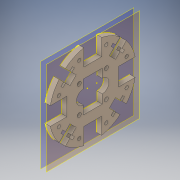
# Autodesk Inventor part: deska
Saved by Autodesk Inventor 2018 (Build 220112000, 112)
## iProperties
Created: 2018-03-10
Part Number: deska
Material: Všeobecné
Document SubType Name: Modeling
Designer: Kuba
Density: 1 g/cm^3
Appearance: Výchozí
Author: Kuba
Autodesk Inventor part; units mm, degrees
ref_plane "YZ Plane" through (0, 0, 0) normal (1, 0, 0) x (0, 1, 0)
ref_plane "XZ Plane" through (0, 0, 0) normal (0, 1, 0) x (-1, 0, 0)
ref_plane "XY Plane" through (0, 0, 0) normal (0, 0, 1) x (1, 0, 0)
sketch "Náčrt1" plane through (0, 0, 0) normal (1, 0, 0) x (0, 1, 0)
  line L0 (19, 6.6) -> (31.312, 6.6)
  line L1 (31.312, -6.6) -> (19, -6.6)
  line L2 (19, -6.6) -> (19, 6.6)
  line L3 (24.8085, 20.2123) -> (16.7938, 12.1976)
  line L4 (16.7938, 12.1976) -> (12.1976, 16.7938)
  line L5 (12.1976, 16.7938) -> (20.2123, 24.8085)
  line L6 (0, 0) -> (14.4957, 14.4957)
  line L7 (6.6, 19) -> (-6.6, 19)
  line L8 (6.6, 31.312) -> (6.6, 19)
  line L9 (-6.6, 19) -> (-6.6, 31.312)
  line L10 (-20.2123, 24.8085) -> (-12.1976, 16.7938)
  line L11 (-12.1976, 16.7938) -> (-16.7938, 12.1976)
  line L12 (-16.7938, 12.1976) -> (-24.8085, 20.2123)
  line L13 (-19, 6.6) -> (-19, -6.6)
  line L14 (-31.312, 6.6) -> (-19, 6.6)
  line L15 (-19, -6.6) -> (-31.312, -6.6)
  line L16 (-24.8085, -20.2123) -> (-16.7938, -12.1976)
  line L17 (-16.7938, -12.1976) -> (-12.1976, -16.7938)
  line L18 (-12.1976, -16.7938) -> (-20.2123, -24.8085)
  line L19 (-6.6, -19) -> (6.6, -19)
  line L20 (-6.6, -31.312) -> (-6.6, -19)
  line L21 (6.6, -19) -> (6.6, -31.312)
  line L22 (20.2123, -24.8085) -> (12.1976, -16.7938)
  line L23 (12.1976, -16.7938) -> (16.7938, -12.1976)
  line L24 (16.7938, -12.1976) -> (24.8085, -20.2123)
  arc A0 (24.8085, -20.2123) -> (31.312, -6.6) centre (0, 0) ccw
  arc A1 (6.6, -31.312) -> (20.2123, -24.8085) centre (0, 0) ccw
  arc A2 (-20.2123, -24.8085) -> (-6.6, -31.312) centre (0, 0) ccw
  arc A3 (-31.312, -6.6) -> (-24.8085, -20.2123) centre (0, 0) ccw
  arc A4 (-24.8085, 20.2123) -> (-31.312, 6.6) centre (0, 0) ccw
  arc A5 (-6.6, 31.312) -> (-20.2123, 24.8085) centre (0, 0) ccw
  arc A6 (31.312, 6.6) -> (24.8085, 20.2123) centre (0, 0) ccw
  arc A7 (20.2123, 24.8085) -> (6.6, 31.312) centre (0, 0) ccw
  line L25 (16.205, 20.8011) -> (20.8011, 16.205)
  line L26 (14.9675, 23.4528) -> (13.5533, 22.0386)
  line L27 (13.5533, 22.0386) -> (22.0386, 13.5533)
  line L28 (22.0386, 13.5533) -> (23.4528, 14.9675)
  line L29 (23.4528, 14.9675) -> (14.9675, 23.4528)
  line L30 (-13.5533, 22.0386) -> (-14.9675, 23.4528)
  line L31 (-22.0386, 13.5533) -> (-13.5533, 22.0386)
  line L32 (-14.9675, 23.4528) -> (-23.4528, 14.9675)
  line L33 (-23.4528, 14.9675) -> (-22.0386, 13.5533)
  line L34 (-22.0386, -13.5533) -> (-23.4528, -14.9675)
  line L35 (-13.5533, -22.0386) -> (-22.0386, -13.5533)
  line L36 (-23.4528, -14.9675) -> (-14.9675, -23.4528)
  line L37 (-14.9675, -23.4528) -> (-13.5533, -22.0386)
  line L38 (13.5533, -22.0386) -> (14.9675, -23.4528)
  line L39 (22.0386, -13.5533) -> (13.5533, -22.0386)
  line L40 (14.9675, -23.4528) -> (23.4528, -14.9675)
  line L41 (23.4528, -14.9675) -> (22.0386, -13.5533)
  point P0 (-14.4957, 14.4957)
  point P1 (-14.4957, -14.4957)
  point P2 (14.4957, -14.4957)
  dimension "d1" = 6.6
  dimension "d2" = 6.6
  dimension "d4" = 6.5
  dimension "d5" = 3.25
  dimension "d6" = 20.5
  dimension "d7" = 45
  dimension "d10" = 360
  dimension "d12" = 2
  dimension "d13" = 12
  dimension "d14" = 1
  dimension "d15" = 2.75
  dimension "d18" = 360
  constraints: 84 end point, 16 point on circle, 8 centre point, 6 midpoint, 4 parallel, 3 perpendicular, 1 coincident, 1 horizontal, 94 other
  measures "d1" vertical distance of point (0, 0) L0.start
  measures "d2" distance from line of point (0, 0) L1
  measures "d4" distance between parallel lines of L3 L5
  measures "d5" distance between parallel lines of L6 L5
  measures "d6" distance from line of point (0, 0) L4
  measures "d7" angle of L2 L6
  measures "d12" distance of L26.start L26.end
  measures "d13" distance of L28.end L26.start
  measures "d14" distance between parallel lines of L25 L29
  measures "d15" distance between parallel lines of L5 L26
extrude "Vysunutí1" add sketch "Náčrt1" along normal mid plane 4 contours L2 L1 A0 L24 L40 L41 L39 L23 L22 L38 A1 L21 L19 L20 A2 L18 L36 L37 L35 L17 L16 L34 A3 L15 L13 L14 A4 L12 L32 L33 L31 L11 L10 L30 A5 L9 L7 L8 A7 L5 L29 L26 L27 L4 L3 L28 A6 L0 | L29 L28 L27 L3 | L5 L27 L26 L29 | L24 L39 L41 L40 | L40 L38 L39 L22 | L32 L30 L31 L10 | L12 L31 L33 L32 | L18 L35 L37 L36 | L36 L34 L35 L16
ref_plane "Pracovní rovina1" through (2, 0, 0) normal (1, 0, 0) x (0, 0, -1)
sketch "Náčrt2" plane through (2, 0, 0) normal (1, 0, 0) x (0, 0, -1)
  line L0 (-6.6, 19) -> (-6.6, 31.312) projected
  arc A0 (-6.6, 31.312) -> (-20.2123, 24.8085) centre (0, 0) ccw projected
  line L1 (-20.2123, 24.8085) -> (-12.1976, 16.7938) projected
  line L2 (-12.1976, 16.7938) -> (-16.7938, 12.1976) projected
  line L3 (-16.7938, 12.1976) -> (-24.8085, 20.2123) projected
  arc A1 (-24.8085, 20.2123) -> (-31.312, 6.6) centre (0, 0) ccw projected
  line L4 (-31.312, 6.6) -> (-19, 6.6) projected
  line L5 (-19, 6.6) -> (-19, -6.6) projected
  line L6 (-19, -6.6) -> (-31.312, -6.6) projected
  arc A2 (-31.312, -6.6) -> (-24.8085, -20.2123) centre (0, 0) ccw projected
  line L7 (-24.8085, -20.2123) -> (-16.7938, -12.1976) projected
  line L8 (-16.7938, -12.1976) -> (-12.1976, -16.7938) projected
  line L9 (-12.1976, -16.7938) -> (-20.2123, -24.8085) projected
  arc A3 (-20.2123, -24.8085) -> (-6.6, -31.312) centre (0, 0) ccw projected
  line L10 (-6.6, -31.312) -> (-6.6, -19) projected
  line L11 (-6.6, -19) -> (6.6, -19) projected
  line L12 (6.6, -19) -> (6.6, -31.312) projected
  arc A4 (6.6, -31.312) -> (20.2123, -24.8085) centre (0, 0) ccw projected
  line L13 (20.2123, -24.8085) -> (12.1976, -16.7938) projected
  line L14 (12.1976, -16.7938) -> (16.7938, -12.1976) projected
  line L15 (16.7938, -12.1976) -> (24.8085, -20.2123) projected
  arc A5 (24.8085, -20.2123) -> (31.312, -6.6) centre (0, 0) ccw projected
  line L16 (31.312, -6.6) -> (19, -6.6) projected
  line L17 (19, -6.6) -> (19, 6.6) projected
  line L18 (19, 6.6) -> (31.312, 6.6) projected
  arc A6 (31.312, 6.6) -> (24.8085, 20.2123) centre (0, 0) ccw projected
  line L19 (24.8085, 20.2123) -> (16.7938, 12.1976) projected
  line L20 (16.7938, 12.1976) -> (12.1976, 16.7938) projected
  line L21 (12.1976, 16.7938) -> (20.2123, 24.8085) projected
  arc A7 (20.2123, 24.8085) -> (6.6, 31.312) centre (0, 0) ccw projected
  line L22 (6.6, 31.312) -> (6.6, 19) projected
  line L23 (6.6, 19) -> (-6.6, 19) projected
  line L24 (-16.7938, 12.1976) -> (-24.8085, 20.2123) projected
  line L25 (-20.8011, 16.205) -> (-16.205, 20.8011)
  line L26 (-23.4528, 14.9675) -> (-14.9675, 23.4528)
  line L27 (-20.2123, 24.8085) -> (-12.1976, 16.7938) projected
  line L28 (-14.9675, 23.4528) -> (-13.5533, 22.0386)
  line L29 (-13.5533, 22.0386) -> (-22.0386, 13.5533)
  line L30 (-22.0386, 13.5533) -> (-23.4528, 14.9675)
  line L31 (-16.205, -20.8011) -> (-20.8011, -16.205)
  line L32 (-22.0386, -13.5533) -> (-13.5533, -22.0386)
  line L33 (-14.9675, -23.4528) -> (-23.4528, -14.9675)
  line L34 (-13.5533, -22.0386) -> (-14.9675, -23.4528)
  line L35 (-23.4528, -14.9675) -> (-22.0386, -13.5533)
  line L36 (20.8011, -16.205) -> (16.205, -20.8011)
  line L37 (13.5533, -22.0386) -> (22.0386, -13.5533)
  line L38 (23.4528, -14.9675) -> (14.9675, -23.4528)
  line L39 (22.0386, -13.5533) -> (23.4528, -14.9675)
  line L40 (14.9675, -23.4528) -> (13.5533, -22.0386)
  line L41 (16.205, 20.8011) -> (20.8011, 16.205)
  line L42 (22.0386, 13.5533) -> (13.5533, 22.0386)
  line L43 (14.9675, 23.4528) -> (23.4528, 14.9675)
  line L44 (13.5533, 22.0386) -> (14.9675, 23.4528)
  line L45 (23.4528, 14.9675) -> (22.0386, 13.5533)
  dimension "d23" = 12
  dimension "d24" = 2
  dimension "d25" = 1
  dimension "d26" = 2.75
  dimension "d27" = 6.5
  dimension "d30" = 360
  constraints: 40 end point, 4 perpendicular, 4 point on line, 2 midpoint, 1 coincident, 49 other
  measures "d23" distance between parallel lines of L30 L28
  measures "d24" distance between parallel lines of L26 L29
  measures "d25" distance between parallel lines of L25 L26
  measures "d26" distance from line of L25.end L28
  measures "d27" distance between parallel lines of L3 L1
extrude "Vysunutí2" cut sketch "Náčrt2" against normal blind 2.5 contours L26 L28 L29 L1 | L1 L25 L3 L26 | L1 L29 L3 L25 | L3 L29 L30 L26 | L43 L19 L41 L21 | L21 L42 L44 L43 | L41 L19 L42 L21 | L43 L45 L42 L19 | L33 L35 L32 L7 | L7 L31 L9 L33 | L7 L32 L9 L31 | L9 L32 L34 L33 | L38 L13 L36 L15 | L15 L37 L39 L38 | L36 L13 L37 L15 | L38 L40 L37 L13
sketch "Náčrt3" plane through (2, 0, 0) normal (1, 0, 0) x (0, 0, -1)
  line L0 (-11.5, 7) -> (-11.5, -7)
  line L1 (11.5, -7) -> (11.5, 7)
  arc A0 (5, 7) -> (-5, 7) centre (0, 7) ccw
  arc A1 (-5, -7) -> (5, -7) centre (0, -7) ccw
  line L2 (-11.5, -7) -> (-5, -7)
  line L3 (5, -7) -> (11.5, -7)
  line L4 (11.5, 7) -> (5, 7)
  line L5 (-5, 7) -> (-11.5, 7)
  point P0 (0, 0)
  dimension "d34" = 23
  dimension "d35" = 14
  dimension "d37" = 11.5
  dimension "d38" = 10
  dimension "d39" = 10
  constraints: 12 end point, 5 parallel, 4 point on circle, 2 centre point, 2 horizontal, 2 perpendicular
  measures "d34" distance of L1.end L0.start
  measures "d35" distance of L0.start L0.end
  measures "d37" distance from line of point (0, 0) L0
  measures "d38" diameter of A0
  measures "d39" diameter of A1
extrude "Vysunutí3" cut sketch "Náčrt3" against normal blind 4
ref_plane "Pracovní rovina2" through (-2, 0, 0) normal (-1, 0, 0) x (0, 0, 1)
sketch "Náčrt4" plane through (-2, 0, 0) normal (-1, 0, 0) x (0, 0, 1)
  line L0 (-11.5, 7) -> (-5, 7) projected
  arc A0 (5, 7) -> (-5, 7) centre (0, 7) ccw projected
  line L1 (5, 7) -> (11.5, 7) projected
  line L2 (11.5, 7) -> (11.5, -7) projected
  line L3 (11.5, -7) -> (5, -7) projected
  arc A1 (-5, -7) -> (5, -7) centre (0, -7) ccw projected
  line L4 (-5, -7) -> (-11.5, -7) projected
  line L5 (-11.5, -7) -> (-11.5, 7) projected
  line L6 (6.6, 31.312) -> (6.6, 19) projected
  line L7 (6.6, 19) -> (-6.6, 19) projected
  line L8 (-6.6, 19) -> (-6.6, 31.312) projected
  arc A2 (-6.6, 31.312) -> (-20.2123, 24.8085) centre (0, 0) ccw projected
  line L9 (-20.2123, 24.8085) -> (-12.1976, 16.7938) projected
  line L10 (-12.1976, 16.7938) -> (-16.7938, 12.1976) projected
  line L11 (-16.7938, 12.1976) -> (-24.8085, 20.2123) projected
  arc A3 (-24.8085, 20.2123) -> (-31.312, 6.6) centre (0, 0) ccw projected
  line L12 (-31.312, 6.6) -> (-19, 6.6) projected
  line L13 (-19, 6.6) -> (-19, -6.6) projected
  line L14 (-19, -6.6) -> (-31.312, -6.6) projected
  arc A4 (-31.312, -6.6) -> (-24.8085, -20.2123) centre (0, 0) ccw projected
  line L15 (-24.8085, -20.2123) -> (-16.7938, -12.1976) projected
  line L16 (-16.7938, -12.1976) -> (-12.1976, -16.7938) projected
  line L17 (-12.1976, -16.7938) -> (-20.2123, -24.8085) projected
  arc A5 (-20.2123, -24.8085) -> (-6.6, -31.312) centre (0, 0) ccw projected
  line L18 (-6.6, -31.312) -> (-6.6, -19) projected
  line L19 (-6.6, -19) -> (6.6, -19) projected
  line L20 (6.6, -19) -> (6.6, -31.312) projected
  arc A6 (6.6, -31.312) -> (20.2123, -24.8085) centre (0, 0) ccw projected
  line L21 (20.2123, -24.8085) -> (12.1976, -16.7938) projected
  line L22 (12.1976, -16.7938) -> (16.7938, -12.1976) projected
  line L23 (16.7938, -12.1976) -> (24.8085, -20.2123) projected
  arc A7 (24.8085, -20.2123) -> (31.312, -6.6) centre (0, 0) ccw projected
  line L24 (31.312, -6.6) -> (19, -6.6) projected
  line L25 (19, -6.6) -> (19, 6.6) projected
  line L26 (19, 6.6) -> (31.312, 6.6) projected
  arc A8 (31.312, 6.6) -> (24.8085, 20.2123) centre (0, 0) ccw projected
  line L27 (24.8085, 20.2123) -> (16.7938, 12.1976) projected
  line L28 (16.7938, 12.1976) -> (12.1976, 16.7938) projected
  line L29 (12.1976, 16.7938) -> (20.2123, 24.8085) projected
  arc A9 (20.2123, 24.8085) -> (6.6, 31.312) centre (0, 0) ccw projected
  line L30 (16.7938, 12.1976) -> (12.1976, 16.7938) projected
  line L31 (-16.7938, -12.1976) -> (-12.1976, -16.7938) projected
sketch "Náčrt5" plane through (-2, 0, 0) normal (-1, 0, 0) x (0, 0, 1)
  circle A0 centre (10, -10) radius 1.5
  circle A1 centre (10, 10) radius 1.5
  circle A2 centre (-10, 10) radius 1.5
  circle A3 centre (-10, -10) radius 1.5
  point P0 (0, 0)
  dimension "d45" = 360
  dimension "d47" = 10
  dimension "d48" = 10
  dimension "d49" = 3
  constraints: 4 centre point, 9 other
  measures "d47" horizontal distance of point (0, 0) A0.centre
  measures "d48" horizontal distance of point (0, 0) A0.centre
  measures "d49" diameter of A0
extrude "Vysunutí4" cut sketch "Náčrt5" against normal blind 4
sketch "Náčrt6" plane through (2, 0, 0) normal (1, 0, 0) x (0, 0, -1)
  circle A0 centre (10, 25) radius 1.25
  circle A1 centre (-10, 25) radius 1.25
  circle A2 centre (-25, 10) radius 1.25
  circle A3 centre (-25, -10) radius 1.25
  circle A4 centre (-10, -25) radius 1.25
  circle A5 centre (10, -25) radius 1.25
  circle A6 centre (25, -10) radius 1.25
  circle A7 centre (25, 10) radius 1.25
  point P0 (0, 0)
  dimension "d52" = 2.5
  dimension "d53" = 2.5
  dimension "d54" = 25
  dimension "d55" = 25
  dimension "d56" = 10
  dimension "d57" = 10
  dimension "d60" = 360
  constraints: 8 centre point, 17 other
  measures "d52" diameter of A0
  measures "d53" diameter of A1
  measures "d54" vertical distance of point (0, 0) A0.centre
  measures "d55" vertical distance of point (0, 0) A1.centre
  measures "d56" horizontal distance of point (0, 0) A0.centre
  measures "d57" horizontal distance of point (0, 0) A1.centre
extrude "Vysunutí5" cut sketch "Náčrt6" against normal blind 4
equation "\"d2\" = d1"
equation "\"d5\" = 0.5 * d4"
equation "\"d14\" = 0.5 * d12"
equation "\"d15\" = -0.5 * d4 + 0.5 * d13"
equation "\"d25\" = 0.5 * d24"
equation "\"d26\" = -0.5 * d27 + 0.5 * d23"
equation "\"d37\" = 0.5 * d34"
equation "\"d39\" = d38"
equation "\"d48\" = d47"
equation "\"d53\" = d52"
equation "\"d55\" = d54"
equation "\"d57\" = d56"
equation "\"d36\" = 0.5 * d35"
